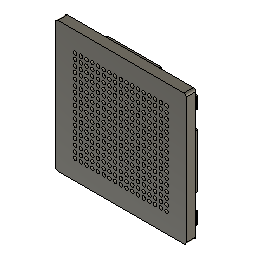
Front_Cover (Autodesk Fusion 360 design; units mm, degrees)
Autodesk Fusion 360 part; units mm, degrees
sketch "Sketch1" plane through (0, 0, 0) normal (0, 1, 0) x (1, 0, 0)
  line L0 (-55, -110) -> (55, -110)
  line L1 (55, -110) -> (55, 0)
  line L2 (55, 0) -> (-55, 0)
  line L3 (-55, 0) -> (-55, -110)
  dimension "width" = 110
  dimension "height" = 110
  constraint horizontal L0
  constraint vertical L1
  constraint horizontal L2
  constraint vertical L3
  constraint midpoint origin L2
  measures "width" distance of L0.start L0.end
  measures "height" distance of L0.end L1.end
extrude "Extrude1" add sketch "Sketch1" along normal blind 2
sketch "Sketch3" plane through (0, 2, 0) normal (0, 1, 0) x (-1, 0, 0)
  line L0 (55, 0) -> (55, 110)
  line L1 (55, 110) -> (-55, 110)
  line L2 (-55, 110) -> (-55, 0)
  line L3 (-55, 0) -> (55, 0)
  line L4 (-55, 110) -> (55, 0) construction
  circle A0 centre (0, 55) radius 50 construction
  line L5 (40, 95) -> (-40, 95)
  line L6 (-40, 95) -> (-40, 15)
  line L7 (-40, 15) -> (40, 15)
  line L8 (40, 15) -> (40, 95)
  circle A1 centre (38.5, 93.5) radius 1.5
  dimension "mesh_cutout_diameter" = 100
  dimension "chime_padding" = 15
  dimension "d23" = 15
  dimension "d24" = 15
  dimension "d25" = 15
  dimension "mesh_hole_diameter" = 3
  constraint coincident L1.end L2.start
  constraint coincident L0.start L3.end
  constraint midpoint L4 A0.centre
  constraint horizontal L5
  constraint vertical L6
  constraint horizontal L7
  constraint vertical L8
  constraint tangent L5 A1
  constraint tangent L8 A1
  measures "mesh_cutout_diameter" diameter of A0
  measures "chime_padding" distance of L0 L8
  measures "d23" distance of L1 L5
  measures "d24" distance of L2 L6
  measures "d25" distance of L3 L7
  measures "mesh_hole_diameter" diameter of A1
extrude "Extrude5" cut sketch "Sketch3" against normal up to surface (2 mm away) contours A1
pattern_linear "R-Pattern1" count 17 spacing 4.8125 along (1, 0, 0) count 17 spacing 4.8125 along (0, 0, -1) of "Extrude5"
sketch "Sketch7" plane through (0, 2, 0) normal (0, 1, 0) x (-1, 0, 0)
  circle A0 centre (-33.6875, 16.5) radius 1.5
  circle A1 centre (-28.875, 16.5) radius 1.5
  circle A2 centre (-24.0625, 16.5) radius 1.5
  circle A3 centre (-19.25, 16.5) radius 1.5
  circle A4 centre (-14.4375, 16.5) radius 1.5
  circle A5 centre (-9.625, 16.5) radius 1.5
  circle A6 centre (-4.8125, 16.5) radius 1.5
  circle A7 centre (0, 16.5) radius 1.5
  circle A8 centre (4.8125, 16.5) radius 1.5
  circle A9 centre (9.625, 16.5) radius 1.5
  circle A10 centre (14.4375, 16.5) radius 1.5
  circle A11 centre (38.5, 16.5) radius 1.5
  circle A12 centre (-38.5, 21.3125) radius 1.5
  circle A13 centre (-33.6875, 21.3125) radius 1.5
  circle A14 centre (-28.875, 21.3125) radius 1.5
  circle A15 centre (-24.0625, 21.3125) radius 1.5
  circle A16 centre (-19.25, 21.3125) radius 1.5
  circle A17 centre (-14.4375, 21.3125) radius 1.5
  circle A18 centre (-9.625, 21.3125) radius 1.5
  circle A19 centre (-4.8125, 21.3125) radius 1.5
  circle A20 centre (0, 21.3125) radius 1.5
  circle A21 centre (4.8125, 21.3125) radius 1.5
  circle A22 centre (9.625, 21.3125) radius 1.5
  circle A23 centre (14.4375, 21.3125) radius 1.5
  circle A24 centre (19.25, 21.3125) radius 1.5
  circle A25 centre (24.0625, 21.3125) radius 1.5
  circle A26 centre (28.875, 21.3125) radius 1.5
  circle A27 centre (33.6875, 21.3125) radius 1.5
  circle A28 centre (38.5, 21.3125) radius 1.5
  circle A29 centre (-38.5, 26.125) radius 1.5
  circle A30 centre (-33.6875, 26.125) radius 1.5
  circle A31 centre (-28.875, 26.125) radius 1.5
  circle A32 centre (-24.0625, 26.125) radius 1.5
  circle A33 centre (-19.25, 26.125) radius 1.5
  circle A34 centre (-14.4375, 26.125) radius 1.5
  circle A35 centre (-9.625, 26.125) radius 1.5
  circle A36 centre (-4.8125, 26.125) radius 1.5
  circle A37 centre (0, 26.125) radius 1.5
  circle A38 centre (4.8125, 26.125) radius 1.5
  circle A39 centre (9.625, 26.125) radius 1.5
  circle A40 centre (14.4375, 26.125) radius 1.5
  circle A41 centre (19.25, 26.125) radius 1.5
  circle A42 centre (24.0625, 26.125) radius 1.5
  circle A43 centre (28.875, 26.125) radius 1.5
  circle A44 centre (33.6875, 26.125) radius 1.5
  circle A45 centre (38.5, 26.125) radius 1.5
  circle A46 centre (-38.5, 30.9375) radius 1.5
  circle A47 centre (-33.6875, 30.9375) radius 1.5
  circle A48 centre (-28.875, 30.9375) radius 1.5
  circle A49 centre (-24.0625, 30.9375) radius 1.5
  circle A50 centre (-19.25, 30.9375) radius 1.5
  circle A51 centre (-14.4375, 30.9375) radius 1.5
  circle A52 centre (-9.625, 30.9375) radius 1.5
  circle A53 centre (-4.8125, 30.9375) radius 1.5
  circle A54 centre (0, 30.9375) radius 1.5
  circle A55 centre (4.8125, 30.9375) radius 1.5
  circle A56 centre (9.625, 30.9375) radius 1.5
  circle A57 centre (14.4375, 30.9375) radius 1.5
  circle A58 centre (19.25, 30.9375) radius 1.5
  circle A59 centre (24.0625, 30.9375) radius 1.5
  circle A60 centre (28.875, 30.9375) radius 1.5
  circle A61 centre (33.6875, 30.9375) radius 1.5
  circle A62 centre (38.5, 30.9375) radius 1.5
  circle A63 centre (-38.5, 35.75) radius 1.5
  circle A64 centre (-33.6875, 35.75) radius 1.5
  circle A65 centre (-28.875, 35.75) radius 1.5
  circle A66 centre (-24.0625, 35.75) radius 1.5
  circle A67 centre (-19.25, 35.75) radius 1.5
  circle A68 centre (-14.4375, 35.75) radius 1.5
  circle A69 centre (-9.625, 35.75) radius 1.5
  circle A70 centre (-4.8125, 35.75) radius 1.5
  circle A71 centre (0, 35.75) radius 1.5
  circle A72 centre (4.8125, 35.75) radius 1.5
  circle A73 centre (9.625, 35.75) radius 1.5
  circle A74 centre (14.4375, 35.75) radius 1.5
  circle A75 centre (19.25, 35.75) radius 1.5
  circle A76 centre (24.0625, 35.75) radius 1.5
  circle A77 centre (28.875, 35.75) radius 1.5
  circle A78 centre (33.6875, 35.75) radius 1.5
  circle A79 centre (38.5, 35.75) radius 1.5
  circle A80 centre (-38.5, 40.5625) radius 1.5
  circle A81 centre (-33.6875, 40.5625) radius 1.5
  circle A82 centre (-28.875, 40.5625) radius 1.5
  circle A83 centre (-24.0625, 40.5625) radius 1.5
  circle A84 centre (-19.25, 40.5625) radius 1.5
  circle A85 centre (-14.4375, 40.5625) radius 1.5
  circle A86 centre (-9.625, 40.5625) radius 1.5
  circle A87 centre (-4.8125, 40.5625) radius 1.5
  circle A88 centre (0, 40.5625) radius 1.5
  circle A89 centre (4.8125, 40.5625) radius 1.5
  circle A90 centre (9.625, 40.5625) radius 1.5
  circle A91 centre (14.4375, 40.5625) radius 1.5
  circle A92 centre (19.25, 40.5625) radius 1.5
  circle A93 centre (24.0625, 40.5625) radius 1.5
  circle A94 centre (28.875, 40.5625) radius 1.5
  circle A95 centre (33.6875, 40.5625) radius 1.5
  circle A96 centre (38.5, 40.5625) radius 1.5
  circle A97 centre (-38.5, 45.375) radius 1.5
  circle A98 centre (-33.6875, 45.375) radius 1.5
  circle A99 centre (-28.875, 45.375) radius 1.5
  circle A100 centre (-24.0625, 45.375) radius 1.5
  circle A101 centre (-19.25, 45.375) radius 1.5
  circle A102 centre (-14.4375, 45.375) radius 1.5
  circle A103 centre (-9.625, 45.375) radius 1.5
  circle A104 centre (-4.8125, 45.375) radius 1.5
  circle A105 centre (0, 45.375) radius 1.5
  circle A106 centre (4.8125, 45.375) radius 1.5
  circle A107 centre (9.625, 45.375) radius 1.5
  circle A108 centre (14.4375, 45.375) radius 1.5
  circle A109 centre (19.25, 45.375) radius 1.5
  circle A110 centre (24.0625, 45.375) radius 1.5
  circle A111 centre (28.875, 45.375) radius 1.5
  circle A112 centre (33.6875, 45.375) radius 1.5
  circle A113 centre (38.5, 45.375) radius 1.5
  circle A114 centre (-38.5, 50.1875) radius 1.5
  circle A115 centre (-33.6875, 50.1875) radius 1.5
  circle A116 centre (-28.875, 50.1875) radius 1.5
  circle A117 centre (-24.0625, 50.1875) radius 1.5
  circle A118 centre (-19.25, 50.1875) radius 1.5
  circle A119 centre (-14.4375, 50.1875) radius 1.5
  circle A120 centre (-9.625, 50.1875) radius 1.5
  circle A121 centre (-4.8125, 50.1875) radius 1.5
  circle A122 centre (0, 50.1875) radius 1.5
  circle A123 centre (4.8125, 50.1875) radius 1.5
  circle A124 centre (9.625, 50.1875) radius 1.5
  circle A125 centre (14.4375, 50.1875) radius 1.5
  circle A126 centre (19.25, 50.1875) radius 1.5
  circle A127 centre (24.0625, 50.1875) radius 1.5
  circle A128 centre (28.875, 50.1875) radius 1.5
  circle A129 centre (33.6875, 50.1875) radius 1.5
  circle A130 centre (38.5, 50.1875) radius 1.5
  circle A131 centre (-38.5, 55) radius 1.5
  circle A132 centre (-33.6875, 55) radius 1.5
  circle A133 centre (-28.875, 55) radius 1.5
  circle A134 centre (-24.0625, 55) radius 1.5
  circle A135 centre (-19.25, 55) radius 1.5
  circle A136 centre (-14.4375, 55) radius 1.5
  circle A137 centre (-9.625, 55) radius 1.5
  circle A138 centre (-4.8125, 55) radius 1.5
  circle A139 centre (0, 55) radius 1.5
  circle A140 centre (4.8125, 55) radius 1.5
  circle A141 centre (9.625, 55) radius 1.5
  circle A142 centre (14.4375, 55) radius 1.5
  circle A143 centre (19.25, 55) radius 1.5
  circle A144 centre (24.0625, 55) radius 1.5
  circle A145 centre (28.875, 55) radius 1.5
  circle A146 centre (33.6875, 55) radius 1.5
  circle A147 centre (38.5, 55) radius 1.5
  circle A148 centre (-38.5, 59.8125) radius 1.5
  circle A149 centre (-33.6875, 59.8125) radius 1.5
  circle A150 centre (-28.875, 59.8125) radius 1.5
  circle A151 centre (-24.0625, 59.8125) radius 1.5
  circle A152 centre (-19.25, 59.8125) radius 1.5
  circle A153 centre (-14.4375, 59.8125) radius 1.5
  circle A154 centre (-9.625, 59.8125) radius 1.5
  circle A155 centre (-4.8125, 59.8125) radius 1.5
  circle A156 centre (0, 59.8125) radius 1.5
  circle A157 centre (4.8125, 59.8125) radius 1.5
  circle A158 centre (9.625, 59.8125) radius 1.5
  circle A159 centre (14.4375, 59.8125) radius 1.5
  circle A160 centre (19.25, 59.8125) radius 1.5
  circle A161 centre (24.0625, 59.8125) radius 1.5
  circle A162 centre (28.875, 59.8125) radius 1.5
  circle A163 centre (33.6875, 59.8125) radius 1.5
  circle A164 centre (38.5, 59.8125) radius 1.5
  circle A165 centre (-38.5, 64.625) radius 1.5
  circle A166 centre (-33.6875, 64.625) radius 1.5
  circle A167 centre (-28.875, 64.625) radius 1.5
  circle A168 centre (-24.0625, 64.625) radius 1.5
  circle A169 centre (-19.25, 64.625) radius 1.5
  circle A170 centre (-14.4375, 64.625) radius 1.5
  circle A171 centre (-9.625, 64.625) radius 1.5
  circle A172 centre (-4.8125, 64.625) radius 1.5
  circle A173 centre (0, 64.625) radius 1.5
  circle A174 centre (4.8125, 64.625) radius 1.5
  circle A175 centre (9.625, 64.625) radius 1.5
  circle A176 centre (14.4375, 64.625) radius 1.5
  circle A177 centre (19.25, 64.625) radius 1.5
  circle A178 centre (24.0625, 64.625) radius 1.5
  circle A179 centre (28.875, 64.625) radius 1.5
  circle A180 centre (33.6875, 64.625) radius 1.5
  circle A181 centre (38.5, 64.625) radius 1.5
  circle A182 centre (-38.5, 69.4375) radius 1.5
  circle A183 centre (-33.6875, 69.4375) radius 1.5
  circle A184 centre (-28.875, 69.4375) radius 1.5
  circle A185 centre (-24.0625, 69.4375) radius 1.5
  circle A186 centre (-19.25, 69.4375) radius 1.5
  circle A187 centre (-14.4375, 69.4375) radius 1.5
  circle A188 centre (-9.625, 69.4375) radius 1.5
  circle A189 centre (-4.8125, 69.4375) radius 1.5
  circle A190 centre (0, 69.4375) radius 1.5
  circle A191 centre (4.8125, 69.4375) radius 1.5
  circle A192 centre (9.625, 69.4375) radius 1.5
  circle A193 centre (14.4375, 69.4375) radius 1.5
  circle A194 centre (19.25, 69.4375) radius 1.5
  circle A195 centre (24.0625, 69.4375) radius 1.5
  circle A196 centre (28.875, 69.4375) radius 1.5
  circle A197 centre (33.6875, 69.4375) radius 1.5
  circle A198 centre (38.5, 69.4375) radius 1.5
  circle A199 centre (-33.6875, 74.25) radius 1.5
  circle A200 centre (-28.875, 74.25) radius 1.5
  circle A201 centre (-24.0625, 74.25) radius 1.5
  circle A202 centre (-19.25, 74.25) radius 1.5
  circle A203 centre (-14.4375, 74.25) radius 1.5
  circle A204 centre (-9.625, 74.25) radius 1.5
  circle A205 centre (-4.8125, 74.25) radius 1.5
  circle A206 centre (0, 74.25) radius 1.5
  circle A207 centre (4.8125, 74.25) radius 1.5
  circle A208 centre (9.625, 74.25) radius 1.5
  circle A209 centre (14.4375, 74.25) radius 1.5
  circle A210 centre (38.5, 74.25) radius 1.5
  circle A211 centre (-33.6875, 79.0625) radius 1.5
  circle A212 centre (-28.875, 79.0625) radius 1.5
  circle A213 centre (-24.0625, 79.0625) radius 1.5
  circle A214 centre (-19.25, 79.0625) radius 1.5
  circle A215 centre (-14.4375, 79.0625) radius 1.5
  circle A216 centre (-9.625, 79.0625) radius 1.5
  circle A217 centre (-4.8125, 79.0625) radius 1.5
  circle A218 centre (0, 79.0625) radius 1.5
  circle A219 centre (4.8125, 79.0625) radius 1.5
  circle A220 centre (9.625, 79.0625) radius 1.5
  circle A221 centre (14.4375, 79.0625) radius 1.5
  circle A222 centre (38.5, 79.0625) radius 1.5
  circle A223 centre (-38.5, 83.875) radius 1.5
  circle A224 centre (-33.6875, 83.875) radius 1.5
  circle A225 centre (-28.875, 83.875) radius 1.5
  circle A226 centre (-24.0625, 83.875) radius 1.5
  circle A227 centre (-19.25, 83.875) radius 1.5
  circle A228 centre (-14.4375, 83.875) radius 1.5
  circle A229 centre (-9.625, 83.875) radius 1.5
  circle A230 centre (-4.8125, 83.875) radius 1.5
  circle A231 centre (0, 83.875) radius 1.5
  circle A232 centre (4.8125, 83.875) radius 1.5
  circle A233 centre (9.625, 83.875) radius 1.5
  circle A234 centre (14.4375, 83.875) radius 1.5
  circle A235 centre (19.25, 83.875) radius 1.5
  circle A236 centre (38.5, 83.875) radius 1.5
  circle A237 centre (-38.5, 88.6875) radius 1.5
  circle A238 centre (-33.6875, 88.6875) radius 1.5
  circle A239 centre (-28.875, 88.6875) radius 1.5
  circle A240 centre (-24.0625, 88.6875) radius 1.5
  circle A241 centre (-19.25, 88.6875) radius 1.5
  circle A242 centre (-14.4375, 88.6875) radius 1.5
  circle A243 centre (-9.625, 88.6875) radius 1.5
  circle A244 centre (-4.8125, 88.6875) radius 1.5
  circle A245 centre (0, 88.6875) radius 1.5
  circle A246 centre (4.8125, 88.6875) radius 1.5
  circle A247 centre (9.625, 88.6875) radius 1.5
  circle A248 centre (14.4375, 88.6875) radius 1.5
  circle A249 centre (19.25, 88.6875) radius 1.5
  circle A250 centre (24.0625, 88.6875) radius 1.5
  circle A251 centre (38.5, 88.6875) radius 1.5
  circle A252 centre (-38.5, 93.5) radius 1.5
  circle A253 centre (-33.6875, 93.5) radius 1.5
  circle A254 centre (-28.875, 93.5) radius 1.5
  circle A255 centre (-24.0625, 93.5) radius 1.5
  circle A256 centre (-19.25, 93.5) radius 1.5
  circle A257 centre (-14.4375, 93.5) radius 1.5
  circle A258 centre (-9.625, 93.5) radius 1.5
  circle A259 centre (-4.8125, 93.5) radius 1.5
  circle A260 centre (0, 93.5) radius 1.5
  circle A261 centre (4.8125, 93.5) radius 1.5
  circle A262 centre (9.625, 93.5) radius 1.5
  circle A263 centre (14.4375, 93.5) radius 1.5
  circle A264 centre (19.25, 93.5) radius 1.5
  circle A265 centre (24.0625, 93.5) radius 1.5
  circle A266 centre (33.6875, 93.5) radius 1.5
  circle A267 centre (38.5, 93.5) radius 1.5
  line L0 (55, 0) -> (55, 110)
  line L1 (55, 110) -> (-55, 110)
  line L2 (-55, 110) -> (-55, 0)
  line L3 (-55, 0) -> (55, 0)
  line L4 (-53, 108) -> (53, 108)
  line L5 (53, 108) -> (53, 2)
  line L6 (53, 2) -> (-53, 2)
  line L7 (-53, 2) -> (-53, 108)
  circle A268 centre (24.0625, 83.875) radius 1.5
  circle A269 centre (-38.5, 16.5) radius 1.5
  circle A270 centre (19.25, 16.5) radius 1.5
  circle A271 centre (-38.5, 74.25) radius 1.5
  circle A272 centre (19.25, 74.25) radius 1.5
  circle A273 centre (-38.5, 79.0625) radius 1.5
  circle A274 centre (19.25, 79.0625) radius 1.5
  circle A275 centre (33.6875, 16.5) radius 1.5
  circle A276 centre (24.0625, 74.25) radius 1.5
  circle A277 centre (28.875, 74.25) radius 1.5
  circle A278 centre (33.6875, 74.25) radius 1.5
  circle A279 centre (24.0625, 79.0625) radius 1.5
  circle A280 centre (28.875, 79.0625) radius 1.5
  circle A281 centre (33.6875, 79.0625) radius 1.5
  circle A282 centre (24.0625, 16.5) radius 1.5
  circle A283 centre (28.875, 16.5) radius 1.5
  circle A284 centre (28.875, 93.5) radius 1.5
  circle A285 centre (28.875, 83.875) radius 1.5
  circle A286 centre (33.6875, 83.875) radius 1.5
  circle A287 centre (28.875, 88.6875) radius 1.5
  circle A288 centre (33.6875, 88.6875) radius 1.5
  dimension "d44" = 2
  dimension "d45" = 2
  dimension "d46" = 2
  dimension "d47" = 2
  constraint horizontal L4
  constraint vertical L5
  constraint horizontal L6
  constraint vertical L7
  measures "d44" distance of L2 L7
  measures "d45" distance of L1 L4
  measures "d46" distance of L0 L5
  measures "d47" distance of L3 L6
extrude "Extrude8" add sketch "Sketch7" along normal blind 6 contours L0 L1 L2 L3
fillet "Fillet1" radius 2 4 edges at (55, 4, 110) (-55, 4, 110) (55, 4, 0) (-55, 4, 0)
fillet "Fillet3" radius 1 4 edges at (53, 5, 108) (-53, 5, 108) (53, 5, 2) (-53, 5, 2)
sketch "Sketch9" plane through (53, 0, 0) normal (-1, 0, 0) x (0, -1, 0)
  line L0 (-8, 3) -> (-2, 3)
  line L1 (-2, 3) -> (-2, 107)
  line L2 (-2, 107) -> (-8, 107)
  line L3 (-8, 107) -> (-8, 3)
  line L4 (-12, 18) -> (-2, 18)
  line L5 (-2, 18) -> (-2, 8)
  line L6 (-2, 8) -> (-12, 8)
  line L7 (-12, 8) -> (-12, 18)
  dimension "d69" = 5
  dimension "d70" = 4
  dimension "d71" = 10
  constraint horizontal L4
  constraint vertical L5
  constraint horizontal L6
  constraint vertical L7
  constraint coincident L1 L4.end
  measures "d69" distance of L0 L6
  measures "d70" distance of L3 L7
  measures "d71" distance of L4.start L6.end
extrude "Extrude10" add sketch "Sketch9" along normal blind 1.5 contours L3 L4 L6 L7 | L1 L3 L4 L5 L6
ref_plane "WorkPlane3" through (0, 4, 55) normal (0, 0, 1) x (1, 0, 0)
ref_plane "WorkPlane4" through (0, 4, 55) normal (1, 0, 0) x (0, 0, -1)
sketch "Sketch11" plane through (0, 0, 8) normal (0, 0, -1) x (1, 0, 0)
  line L0 (53, -8) -> (53, -2)
  line L1 (53, -2) -> (51.5, -2)
  line L2 (51.5, -2) -> (51.5, -12)
  line L3 (51.5, -12) -> (53, -12)
  line L4 (53, -12) -> (53, -8)
  line L5 (-53, 0) -> (-53, -8)
  line L6 (-53, -8) -> (53, -8)
  line L7 (53, -8) -> (53, 0)
  line L8 (53, 0) -> (-53, 0)
  line L9 (53, -11.05) -> (51.9, -11.05)
  line L10 (51.9, -11.05) -> (51.9, -8)
  line L11 (51.9, -8) -> (53, -8)
  line L12 (53, -8) -> (53, -11.05)
  dimension "d86" = 1.1
  dimension "d90" = 0.95
  constraint horizontal L9
  constraint vertical L10
  constraint horizontal L11
  constraint vertical L12
  constraint coincident L4 L9.start
  constraint coincident L0.start L11
  measures "d86" distance of L9.start L9.end
  measures "d90" distance of L3 L9
extrude "Extrude12" cut sketch "Sketch11" against normal up to surface (10 mm away) contours L4 L6 L9 L10 L11 L12
fillet "Fillet5" radius 1 1 edges at (51.9, 8, 13)
chamfer "Chamfer1" distance 0.75 angle 45 1 edges at (53, 12, 13)
mirror "Mirror8" about plane through (0, 4, 55) normal (1, 0, 0) of "Extrude10", "Extrude12", "Fillet5", "Chamfer1"
mirror "Mirror9" about plane through (0, 4, 55) normal (0, 0, 1) of "Extrude10", "Extrude12", "Fillet5", "Chamfer1"
mirror "Mirror10" about plane through (0, 4, 55) normal (1, 0, 0) of "Mirror9"
sketch "Sketch12" plane through (53, 0, 0) normal (-1, 0, 0) x (0, -1, 0)
  line L0 (-2, 92) -> (-8, 92)
  line L1 (-8, 92) -> (-8, 18)
  line L2 (-8, 18) -> (-2, 18)
  line L3 (-2, 18) -> (-2, 92)
  line L4 (-12, 8) -> (-2, 8)
  line L5 (-2, 8) -> (-2, 18)
  line L6 (-2, 18) -> (-12, 18)
  line L7 (-12, 18) -> (-12, 8)
  line L8 (-12, 77.5) -> (-2, 77.5)
  line L9 (-2, 77.5) -> (-2, 32.5)
  line L10 (-2, 32.5) -> (-12, 32.5)
  line L11 (-12, 32.5) -> (-12, 77.5)
  line L12 (-8, 55) -> (-2, 55) construction
  dimension "d100" = 45
  constraint horizontal L8
  constraint vertical L9
  constraint horizontal L10
  constraint vertical L11
  constraint midpoint L1 L12.start
  constraint midpoint L3 L12.end
  constraint coincident L9 L12.end
  constraint midpoint L9 L12.end
  constraint coincident L6.end L11
  measures "d100" distance of L8.start L10.end
extrude "Extrude13" add sketch "Sketch12" along normal up to surface (1.5 mm away) contours L1 L3 L8 L9 L10 | L1 L8 L10 L11
chamfer "Chamfer2" distance 0.5 angle 45 1 edges at (53, 12, 55)
pattern_circular "C-Pattern1" count 4 over 360 about axis through (0, 10.72, 55) along (0, -1, 0) of "Extrude13", "Chamfer2"
equation "width = chime_width"
equation "height = chime_height"
equation "wall_thickness = chime_wall_thickness"
equation "mesh_thickness = 1 mm"
equation "d23 = chime_padding"
equation "d24 = chime_padding"
equation "d25 = chime_padding"
equation "d31 = width - ( chime_padding * 2 ) - mesh_hole_diameter"
equation "d32 = height - ( chime_padding * 2 ) - mesh_hole_diameter"
equation "d44 = wall_thickness"
equation "d45 = d44"
equation "d46 = d44"
equation "d47 = d44"
equation "overlap_height = 6 mm"
equation "speaker_riser_height = 5 mm"
equation "chime_width = 110 mm"
equation "chime_height = 110 mm"
equation "chime_wall_thickness = 2 mm"
named bodies: "Chime_Front_Cover"
